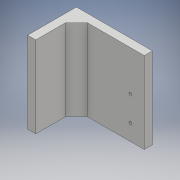
# Autodesk Inventor part: Estrutura - SensorX
Saved by Autodesk Inventor 2017 (Build 210142000, 142)
## iProperties
Created: 2020-09-29
Part Number: Estrutura - SensorX
Material: Generic
Document SubType Name: Modeling
Designer: ale
Density: 1 g/cm^3
Appearance: Default
Author: ale
Autodesk Inventor part; units mm, degrees
ref_plane "YZ Plane" through (0, 0, 0) normal (1, 0, 0) x (0, 1, 0)
ref_plane "XZ Plane" through (0, 0, 0) normal (0, 1, 0) x (-1, 0, 0)
ref_plane "XY Plane" through (0, 0, 0) normal (0, 0, 1) x (1, 0, 0)
sketch "Sketch1" plane through (0, 0, 0) normal (0, 0, 1) x (1, 0, 0)
  line L0 (0, -4) -> (0, -15)
  line L1 (4, 0) -> (25, 0)
  line L2 (25, 3) -> (-3, 3)
  line L3 (-3, 3) -> (-3, -15)
  line L4 (25, 3) -> (25, 0)
  line L5 (0, -15) -> (-3, -15)
  line L6 (4, 0) -> (0, -4)
  point P0 (0, 0)
  point P1 (0, 0)
  dimension "d0" = 15
  dimension "d1" = 25
  dimension "d2" = 3
  dimension "d5" = 4
  dimension "d6" = 4
  constraints: 14 end point, 4 point on line, 2 vertical, 1 horizontal, 1 perpendicular, 1 other
  measures "d0" distance of point (0, 0) L0.end
  measures "d1" distance of point (0, 0) L1.end
  measures "d2" distance between parallel lines of L1 L2
  measures "d5" distance of L1.start point (0, 0)
  measures "d6" distance of L0.start point (0, 0)
extrude "Extrusion1" add sketch "Sketch1" along normal blind 30
sketch "Sketch2" plane through (-3, 3, 0) normal (0, 1, 0) x (1, 0, 0)
  line L0 (28, 0) -> (0, 0) projected
  line L1 (28, 0) -> (28, -30) projected
  point P0 (3, 0)
  point P1 (23, -6)
  point P2 (23, -15.2)
  dimension "d9" = 9.2
  dimension "d10" = 6
  dimension "d11" = 5
  dimension "d12" = 5
  measures "d9" distance of point (23, -15.2) point (23, -6)
  measures "d10" distance from line of point (23, -6) L0
  measures "d11" distance from line of point (23, -6) L1
  measures "d12" distance from line of L1 point (23, -15.2)
hole "Hole1" at (20, 3, 6) at (20, 3, 15.2) direction (0, -1, 0) diameter 1 end through all
equation "\"d6\" = d5"
body "Solid1"
